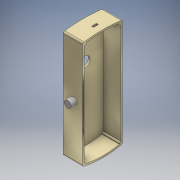
# Autodesk Inventor part: ET11
Saved by Autodesk Inventor 2016 (Build 200138000, 138)
## iProperties
Created: 2016-03-20
Part Number: ET11
Material: Genérico
Document SubType Name: Modeling
Designer: Usuario1
Density: 1 g/cm^3
Appearance: Valor por defecto
Author: Usuario1
Autodesk Inventor part; units mm, degrees
ref_plane "YZ Plane" through (0, 0, 0) normal (1, 0, 0) x (0, 1, 0)
ref_plane "XZ Plane" through (0, 0, 0) normal (0, 1, 0) x (-1, 0, 0)
sketch "Boceto1" plane through (0, 0, 0) normal (1, 0, 0) x (0, 1, 0)
  line L0 (-0.15, 0.1285) -> (-0.15, 8.6735)
  line L1 (-0.16, 0.1285) -> (-0.15, 0.1285)
  arc A0 (-0.16, 0.1285) -> (-0.28, 0.0085) centre (-0.16, 0.0085) ccw
  line L2 (-0.28, -0.0286) -> (-0.28, 0.0085)
  arc A1 (-3.1278, -0.0286) -> (-0.28, -0.0286) centre (-1.7039, 6.7442) ccw
  line L3 (-3.1278, 0.0085) -> (-3.1278, -0.0286)
  arc A2 (-3.1278, 0.0085) -> (-3.2478, 0.1285) centre (-3.2478, 0.0085) ccw
  line L4 (-3.2578, 0.1285) -> (-3.2478, 0.1285)
  line L5 (-3.2578, 8.6735) -> (-3.2578, 0.1285)
  line L6 (-3.2578, 8.6735) -> (-3.1978, 8.6735)
  arc A3 (-3.1978, 8.6735) -> (-3.07, 8.818) centre (-3.2478, 8.8464) ccw
  line L7 (-3.07, 8.818) -> (-3.0698, 8.8784)
  arc A4 (-0.3377, 8.8784) -> (-3.0698, 8.8784) centre (-1.7039, -2.8031) ccw
  line L8 (-0.3377, 8.8784) -> (-0.3377, 8.818)
  arc A5 (-0.3377, 8.818) -> (-0.21, 8.6735) centre (-0.16, 8.8464) ccw
  line L9 (-0.21, 8.6735) -> (-0.15, 8.6735)
  line L10 (0, 8.8549) -> (0, 0)
  arc A6 (0, 8.8549) -> (-0.1302, 9.0036) centre (-0.15, 8.8549) ccw
  arc A7 (-0.1302, 9.0036) -> (-3.2776, 9.0036) centre (-1.7039, -2.8031) ccw
  arc A8 (-3.2776, 9.0036) -> (-3.4078, 8.8549) centre (-3.2578, 8.8549) ccw
  line L11 (-3.4078, 8.7264) -> (-3.4078, 8.8549)
  line L12 (-3.4078, 0.1285) -> (-3.4078, 8.7264)
  line L13 (-3.4078, 0) -> (-3.4078, 0.1285)
  arc A9 (-3.4078, 0) -> (-3.2914, -0.1462) centre (-3.2578, 0) ccw
  arc A10 (-3.2914, -0.1462) -> (-0.28, -0.1818) centre (-1.7039, 6.7442) ccw
  arc A11 (-0.28, -0.1818) -> (-0.1163, -0.1462) centre (-1.7039, 6.7442) ccw
  arc A12 (-0.1163, -0.1462) -> (0, 0) centre (-0.15, 0) ccw
  point P0 (0, 0)
  point P1 (0, 0)
  constraints: 28 end point, 26 point on circle, 13 centre point
extrude "Extrusión1" add sketch "Boceto1" along normal blind 0.75
sketch "Boceto2" plane through (0, 0, 0) normal (-1, 0, 0) x (0, 0, 1)
  line L0 (0.1285, -0.16) -> (0.1285, -0.15) projected
  line L1 (0.1285, -0.15) -> (8.6735, -0.15) projected
  line L2 (8.6735, -0.15) -> (8.6735, -0.21) projected
  arc A0 (8.6735, -0.21) -> (8.818, -0.3377) centre (8.8464, -0.16) ccw projected
  line L3 (8.818, -0.3377) -> (8.8784, -0.3377) projected
  arc A1 (8.8784, -3.0698) -> (8.8784, -0.3377) centre (-2.8031, -1.7039) ccw projected
  line L4 (8.8784, -3.0698) -> (8.818, -3.07) projected
  arc A2 (8.818, -3.07) -> (8.6735, -3.1978) centre (8.8464, -3.2478) ccw projected
  line L5 (8.6735, -3.1978) -> (8.6735, -3.2578) projected
  line L6 (8.6735, -3.2578) -> (0.1285, -3.2578) projected
  line L7 (0.1285, -3.2578) -> (0.1285, -3.2478) projected
  arc A3 (0.1285, -3.2478) -> (0.0085, -3.1278) centre (0.0085, -3.2478) ccw projected
  line L8 (0.0085, -3.1278) -> (-0.0286, -3.1278) projected
  arc A4 (-0.0286, -0.28) -> (-0.0286, -3.1278) centre (6.7442, -1.7039) ccw projected
  line L9 (-0.0286, -0.28) -> (0.0085, -0.28) projected
  arc A5 (0.0085, -0.28) -> (0.1285, -0.16) centre (0.0085, -0.16) ccw projected
  line L10 (8.8549, 0) -> (0, 0) projected
  arc A6 (0, 0) -> (-0.1462, -0.1163) centre (0, -0.15) ccw projected
  arc A7 (-0.1462, -0.1163) -> (-0.1818, -0.28) centre (6.7442, -1.7039) ccw projected
  arc A8 (-0.1818, -0.28) -> (-0.1462, -3.2914) centre (6.7442, -1.7039) ccw projected
  arc A9 (-0.1462, -3.2914) -> (0, -3.4078) centre (0, -3.2578) ccw projected
  line L11 (0, -3.4078) -> (8.8549, -3.4078) projected
  arc A10 (8.8549, -3.4078) -> (9.0036, -3.2776) centre (8.8549, -3.2578) ccw projected
  arc A11 (9.0036, -3.2776) -> (9.0036, -0.1302) centre (-2.8031, -1.7039) ccw projected
  arc A12 (9.0036, -0.1302) -> (8.8549, 0) centre (8.8549, -0.15) ccw projected
  point P0 (0, 0)
extrude "Extrusión2" add sketch "Boceto2" along normal blind 0.88
sketch "Boceto3" plane through (-0.88, 0, 0) normal (-1, 0, 0) x (0, 0, 1)
  line L0 (0.1285, -0.15) -> (8.6735, -0.15) projected
  line L1 (8.6735, -0.15) -> (8.6735, -0.21) projected
  arc A0 (8.6735, -0.21) -> (8.818, -0.3377) centre (8.8464, -0.16) ccw projected
  line L2 (8.818, -0.3377) -> (8.8784, -0.3377) projected
  arc A1 (8.8784, -3.0698) -> (8.8784, -0.3377) centre (-2.8031, -1.7039) ccw projected
  line L3 (8.8784, -3.0698) -> (8.818, -3.07) projected
  arc A2 (8.818, -3.07) -> (8.6735, -3.1978) centre (8.8464, -3.2478) ccw projected
  line L4 (8.6735, -3.1978) -> (8.6735, -3.2578) projected
  line L5 (8.6735, -3.2578) -> (0.1285, -3.2578) projected
  line L6 (0.1285, -3.2578) -> (0.1285, -3.2478) projected
  arc A3 (0.1285, -3.2478) -> (0.0085, -3.1278) centre (0.0085, -3.2478) ccw projected
  line L7 (0.0085, -3.1278) -> (-0.0286, -3.1278) projected
  arc A4 (-0.0286, -0.28) -> (-0.0286, -3.1278) centre (6.7442, -1.7039) ccw projected
  line L8 (-0.0286, -0.28) -> (0.0085, -0.28) projected
  arc A5 (0.0085, -0.28) -> (0.1285, -0.16) centre (0.0085, -0.16) ccw projected
  line L9 (0.1285, -0.16) -> (0.1285, -0.15) projected
  line L10 (8.8549, 0) -> (0, 0) projected
  arc A6 (0, 0) -> (-0.1462, -0.1163) centre (0, -0.15) ccw projected
  arc A7 (-0.1462, -0.1163) -> (-0.1818, -0.28) centre (6.7442, -1.7039) ccw projected
  arc A8 (-0.1818, -0.28) -> (-0.1462, -3.2914) centre (6.7442, -1.7039) ccw projected
  arc A9 (-0.1462, -3.2914) -> (0, -3.4078) centre (0, -3.2578) ccw projected
  line L11 (0, -3.4078) -> (8.8549, -3.4078) projected
  arc A10 (8.8549, -3.4078) -> (9.0036, -3.2776) centre (8.8549, -3.2578) ccw projected
  arc A11 (9.0036, -3.2776) -> (9.0036, -0.1302) centre (-2.8031, -1.7039) ccw projected
  arc A12 (9.0036, -0.1302) -> (8.8549, 0) centre (8.8549, -0.15) ccw projected
  point P0 (0, 0)
extrude "Extrusión3" add sketch "Boceto3" against normal blind 0.15 contours L0 L1 A0 L2 A1 L3 A2 L4 L5 L6 A3 L7 A4 L8 A5 L9
sketch "Boceto4" plane through (-0.88, 0, 0) normal (-1, 0, 0) x (0, 0, 1)
  circle A0 centre (6.008, -1.7039) radius 0.225
  line L0 (8.8549, 0) -> (0, 0)
  arc A1 (0, 0) -> (-0.1462, -0.1163) centre (0, -0.15) ccw
  arc A2 (-0.1462, -0.1163) -> (-0.1462, -3.2914) centre (6.7442, -1.7039) ccw
  arc A3 (-0.1462, -3.2914) -> (0, -3.4078) centre (0, -3.2578) ccw
  line L1 (0, -3.4078) -> (8.8549, -3.4078)
  arc A4 (8.8549, -3.4078) -> (9.0036, -3.2776) centre (8.8549, -3.2578) ccw
  arc A5 (9.0036, -3.2776) -> (9.0036, -0.1302) centre (-2.8031, -1.7039) ccw
  arc A6 (9.0036, -0.1302) -> (8.8549, 0) centre (8.8549, -0.15) ccw
  line L2 (8.8549, 0) -> (0, 0) projected
  arc A7 (0, 0) -> (-0.1462, -0.1163) centre (0, -0.15) ccw projected
  arc A8 (-0.1462, -0.1163) -> (-0.1818, -0.28) centre (6.7442, -1.7039) ccw projected
  arc A9 (-0.1818, -0.28) -> (-0.1462, -3.2914) centre (6.7442, -1.7039) ccw projected
  arc A10 (-0.1462, -3.2914) -> (0, -3.4078) centre (0, -3.2578) ccw projected
  line L3 (0, -3.4078) -> (8.8549, -3.4078) projected
  arc A11 (8.8549, -3.4078) -> (9.0036, -3.2776) centre (8.8549, -3.2578) ccw projected
  arc A12 (9.0036, -3.2776) -> (9.0036, -0.1302) centre (-2.8031, -1.7039) ccw projected
  arc A13 (9.0036, -0.1302) -> (8.8549, 0) centre (8.8549, -0.15) ccw projected
  circle A14 centre (6.008, -1.7039) radius 0.425
  point P0 (0, 0)
  point P1 (-0.1818, -0.28)
  dimension "d11" = 0.85
  constraints: 12 point on circle, 8 centre point, 4 end point, 1 coincident
  measures "d11" diameter of A14
extrude "Extrusión4" cut sketch "Boceto4" against normal blind 10 contours A0 | A14
ref_plane "Plano de trabajo1" through (0, 0, 9.11) normal (0, 0, 1) x (1, 0, 0)
sketch "Boceto5" plane through (0, 0, 9.11) normal (0, 0, 1) x (1, 0, 0)
  line L0 (0.75, -3.2776) -> (0.75, -0.1302) projected
  line L1 (-0.88, -2.1289) -> (-0.88, -1.2789) projected
  line L2 (0.197, -1.9139) -> (0.197, -1.4939)
  line L3 (0.197, -1.4939) -> (0.027, -1.4939)
  line L4 (0.027, -1.4939) -> (0.027, -1.9139)
  line L5 (0.197, -1.9139) -> (0.027, -1.9139)
  line L6 (0.75, -3.4078) -> (-0.88, -3.4078) projected
  point P0 (0, 0)
  dimension "d14" = 0.42
  dimension "d15" = 0.17
  constraints: 8 end point, 1 perpendicular
  measures "d14" distance of L2.start L2.end
  measures "d15" distance of L2.end L3.end
extrude "Extrusión5" cut sketch "Boceto5" against normal blind 1
sketch "Boceto6" plane through (0.75, -3.4078, 0) normal (0, -1, 0) x (1, 0, 0)
  line L0 (0, 0) -> (-1.63, 0) projected
  line L1 (0, 8.8549) -> (0, 0) projected
  line L2 (0, 8.8549) -> (-1.63, 8.8549) projected
  line L3 (-1.63, 0) -> (-1.63, 8.8549) projected
  line L4 (-1.63, 0) -> (-1.63, 8.8549) projected
  line L5 (-1.63, 8.8549) -> (-1.63, 0)
  line L6 (-0.75, 8.8549) -> (-0.75, 0)
  line L7 (-0.75, 0) -> (-0.75, 4.35)
  circle A0 centre (-0.75, 4.35) radius 0.3
  point P0 (-0.75, 0)
  dimension "d18" = 4.35
  dimension "d19" = 0.6
  constraints: 6 end point, 2 vertical, 1 centre point, 1 coincident, 1 point on line
  measures "d18" distance of L6.end L7.end
  measures "d19" diameter of A0
extrude "Extrusión6" add sketch "Boceto6" along normal blind 0.5 contours A0 L6 | L6 A0
